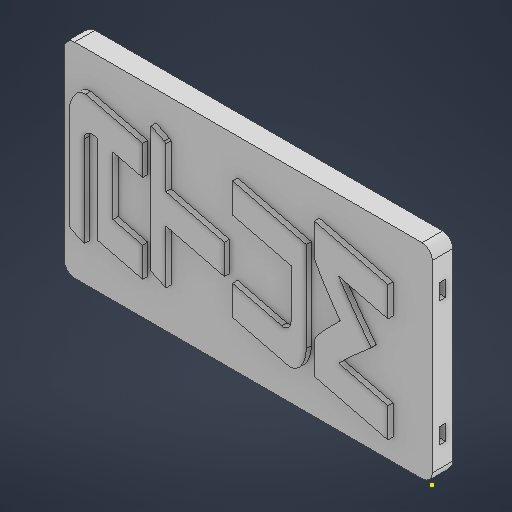
# Autodesk Inventor part: custom  plate vertical
Saved by Autodesk Inventor 2025.1 (Build 291241000, 241)
## iProperties
Created: 2024-12-05
Part Number: custom  plate vertical
Material: Generic
Document SubType Name: Modeling
Designer: Hunter Mathis
Density: 1 g/cm^3
Appearance: Default
Author: Hunter Mathis
Autodesk Inventor part; units mm, degrees
ref_plane "YZ Plane" through (0, 0, 0) normal (1, 0, 0) x (0, 1, 0)
ref_plane "XZ Plane" through (0, 0, 0) normal (0, 1, 0) x (-1, 0, 0)
sketch "Sketch1" plane through (0, 0, 0) normal (0, 0, 1) x (1, 0, 0)
  line L0 (0, 0) -> (-114.3, 0)
  line L1 (-114.3, 0) -> (-114.3, 63.5)
  line L2 (-114.3, 63.5) -> (0, 63.5)
  line L3 (0, 63.5) -> (0, 0)
  dimension "d7" = 114.3
  dimension "d8" = 63.5
  constraints: 8 end point, 2 parallel, 1 horizontal, 1 perpendicular
  measures "d7" distance of L1.end L2.end
  measures "d8" distance of L0.end L1.end
extrude "Extrusion1" add sketch "Sketch1" along normal blind 6.35
sketch "Sketch2" plane through (0, 0, 6.35) normal (0, 0, 1) x (1, 0, 0)
  line L0 (0, 0) -> (0, 63.5) projected
  line L1 (-114.3, 63.5) -> (-114.3, 0) projected
  line L2 (-114.3, 0) -> (0, 0) projected
  line L3 (0, 63.5) -> (-114.3, 63.5) projected
sketch "Sketch3" plane through (0, 0, 6.35) normal (0, 0, 1) x (1, 0, 0)
  line L0 (-110.6716, 35.2666) -> (-52.0005, 35.2666) construction
  line L1 (-52.0005, 35.2666) -> (-52.0005, 28.3217) construction
  line L2 (-52.0005, 28.3217) -> (-110.6716, 28.3217) construction
  line L3 (-110.6716, 28.3217) -> (-110.6716, 35.2666) construction
  line L4 (-114.3, 63.5) -> (-114.3, 0) projected
  point P0 (0, 0)
  constraints: 2 other
extrude "Extrusion2" [suppressed]
fillet "Fillet2" radius 3.175 4 edges at (-114.3, 63.5, 3.175) (-114.3, 0, 3.175) (0, 0, 3.175) (0, 63.5, 3.175)
sketch "Sketch4" plane through (0, 0, 6.35) normal (0, 0, 1) x (1, 0, 0)
  point P0 (0, 0)
sketch "Sketch5" plane through (0, 0, 6.35) normal (0, 0, 1) x (1, 0, 0)
  point P0 (0, 0)
sketch "Sketch6" plane through (0, 0, 6.35) normal (0, 0, 1) x (1, 0, 0)
  point P0 (0, 0)
ref_plane "Work Plane1" through (-57.15, 3.175, 0) normal (1, 0, 0) x (0, 0, -1)
sketch "Sketch7" plane through (-111.125, 63.5, 0) normal (0, 1, 0) x (1, 0, 0)
  line L0 (107.95, -6.35) -> (0, -6.35) projected
  line L1 (107.95, 0) -> (0, 0) projected
  line L2 (0, -6.35) -> (0, -3.175)
  line L3 (0, -6.35) -> (0, 0) projected
  line L4 (0, 0) -> (0, -6.35) projected
  line L5 (0, -6.35) -> (0, -3.5306)
  line L6 (0, -3.5306) -> (6.985, -3.5306)
  line L7 (6.985, -3.5306) -> (11.8618, -3.5306)
  line L8 (11.8618, -3.5306) -> (11.8618, -1.651)
  line L9 (11.8618, -1.651) -> (6.985, -1.651)
  line L10 (6.985, -1.651) -> (6.985, -3.5306)
  point P0 (111.125, 0)
  dimension "d24" = 4.8768
  dimension "d25" = 1.8796
  dimension "d26" = 2.8194
  dimension "d27" = 6.985
  constraints: 14 end point, 2 horizontal, 2 parallel, 1 midpoint, 1 perpendicular, 1 point on line
  measures "d24" distance of L6.end L7.end
  measures "d25" distance of L7.end L8.end
  measures "d26" distance between parallel lines of L6 L0
  measures "d27" distance of L5.end L6.end
extrude "Extrusion3" [suppressed]
sketch "Sketch8" plane through (-111.125, 0, 0) normal (0, -1, 0) x (1, 0, 0)
  line L0 (0, 0) -> (0, 6.35) projected
  line L1 (6.985, 3.5306) -> (6.985, 1.651) projected
  line L2 (11.8618, 1.651) -> (11.8618, 3.5306) projected
  line L3 (6.985, 1.651) -> (11.8618, 1.651)
  line L4 (11.8618, 1.651) -> (11.8618, 3.5306)
  line L5 (11.8618, 3.5306) -> (6.985, 3.5306)
  line L6 (6.985, 3.5306) -> (6.985, 1.651)
  line L7 (0, 0) -> (107.95, 0) projected
  point P0 (111.125, 0)
  constraints: 8 end point, 2 parallel, 1 horizontal, 1 perpendicular
extrude "Extrusion4" [suppressed]
mirror "Mirror1" [suppressed]
mirror "Mirror2" [suppressed]
sketch "Sketch9" plane through (0, 0, 6.35) normal (0, 0, 1) x (1, 0, 0)
  point P0 (0, 0)
sketch "Sketch10" plane through (0, 0, 6.35) normal (0, 0, 1) x (1, 0, 0)
  line L0 (-111.2518, 27.0157) -> (-111.2518, 30.2464) construction
  line L1 (-111.2518, 30.2464) -> (-93.1484, 30.2464) construction
  line L2 (-93.1484, 30.2464) -> (-93.1484, 27.0157) construction
  line L3 (-93.1484, 27.0157) -> (-111.2518, 27.0157) construction
  line L4 (-114.3, 60.325) -> (-114.3, 3.175) projected
  line L5 (-114.3, 60.325) -> (-114.3, 3.175)
  line L6 (-114.3, 3.175) -> (-114.3, 31.75)
  line L7 (0, 3.175) -> (0, 60.325) projected
  line L8 (-88.3918, 11.8288) -> (-102.3042, 15.3115)
  line L9 (-102.3042, 15.3115) -> (-102.3042, 42.6731)
  line L10 (-102.3042, 42.6731) -> (-103.638, 42.988)
  spline S0 degree 2 poles (-103.638, 42.988) (-104.2308, 43.1362) (-105.2867, 42.8213) (-106.0833, 42.1173) (-106.5464, 41.0799) (-106.5464, 40.5242) knots 0 0 0 1 2 3 4 4 4
  line L11 (-106.5464, 40.5242) -> (-106.5464, 12.3845)
  spline S1 degree 2 poles (-106.5464, 12.3845) (-107.4912, 12.8106) (-109.7327, 13.8295) (-110.6775, 14.3297) knots 0 0 0 1 2 2 2
  line L12 (-110.6775, 14.3297) -> (-111.2518, 14.7743)
  line L13 (-111.2518, 14.7743) -> (-111.2518, 45.3222)
  spline S2 degree 2 poles (-111.2518, 45.3222) (-111.2518, 46.5078) (-110.6034, 49.1569) (-109.2881, 51.3984) (-107.38, 52.8434) (-106.0648, 52.8063) knots 0 0 0 1 2 3 4 4 4
  line L14 (-106.0648, 52.8063) -> (-88.3918, 48.3974)
  line L15 (-88.3918, 48.3974) -> (-88.3918, 39.1904)
  line L16 (-88.3918, 39.1904) -> (-97.5988, 41.469)
  line L17 (-97.5988, 41.469) -> (-97.5988, 23.3143)
  line L18 (-97.5988, 23.3143) -> (-88.3918, 21.0358)
  line L19 (-88.3918, 21.0358) -> (-88.3918, 11.8288)
  spline S3 degree 2 poles (-81.1464, 13.144) (-82.0912, 13.5701) (-84.3327, 14.589) (-85.2775, 15.0892) knots 0 0 0 1 2 2 2
  line L20 (-85.2775, 15.0892) -> (-85.8518, 15.5338)
  line L21 (-85.8518, 15.5338) -> (-85.8518, 54.3439)
  spline S4 degree 2 poles (-85.8518, 54.3439) (-84.907, 53.9734) (-82.6655, 52.9175) (-81.7207, 52.3803) knots 0 0 0 1 2 2 2
  line L22 (-81.7207, 52.3803) -> (-81.1464, 51.9357)
  line L23 (-81.1464, 51.9357) -> (-81.1464, 39.0051)
  line L24 (-81.1464, 39.0051) -> (-62.9918, 34.485)
  line L25 (-62.9918, 34.485) -> (-62.9918, 25.278)
  line L26 (-62.9918, 25.278) -> (-81.1464, 29.7981)
  line L27 (-81.1464, 29.7981) -> (-81.1464, 13.144)
  spline S5 degree 2 poles (-42.7788, 11.1619) (-41.4635, 11.1248) (-39.5555, 12.5512) (-38.2402, 14.7928) (-37.5918, 17.4419) (-37.5918, 18.6275) knots 0 0 0 1 2 3 4 4 4
  line L28 (-37.5918, 18.6275) -> (-37.5918, 46.6004)
  line L29 (-37.5918, 46.6004) -> (-60.4518, 52.2876)
  line L30 (-60.4518, 52.2876) -> (-60.4518, 43.0806)
  line L31 (-60.4518, 43.0806) -> (-42.2972, 38.5605)
  line L32 (-42.2972, 38.5605) -> (-42.2972, 23.407)
  spline S6 degree 2 poles (-42.2972, 23.407) (-42.2972, 22.8697) (-42.7603, 21.8509) (-43.5569, 21.1284) (-44.6128, 20.8134) (-45.1871, 20.9431) knots 0 0 0 1 2 3 4 4 4
  line L33 (-45.1871, 20.9431) -> (-60.4518, 24.7593)
  line L34 (-60.4518, 24.7593) -> (-60.4518, 15.5523)
  line L35 (-60.4518, 15.5523) -> (-42.7788, 11.1619)
  line L36 (-35.0518, 12.403) -> (-12.1918, 6.7158)
  line L37 (-12.1918, 6.7158) -> (-12.1918, 15.9228)
  line L38 (-12.1918, 15.9228) -> (-27.475, 19.7205)
  spline S7 degree 2 poles (-27.475, 19.7205) (-26.5302, 20.7393) (-24.1775, 22.9809) (-21.5655, 25.3336) (-18.8238, 27.6863) (-17.4715, 28.8534) knots 0 0 0 1 2 3 4 4 4
  line L39 (-17.4715, 28.8534) -> (-17.4715, 28.9645)
  spline S8 degree 2 poles (-17.4715, 28.9645) (-18.8238, 30.78) (-21.6026, 34.5406) (-24.2146, 38.1715) (-26.5302, 41.5986) (-27.475, 43.0992) knots 0 0 0 1 2 3 4 4 4
  line L40 (-27.475, 43.0992) -> (-12.1918, 39.283)
  line L41 (-12.1918, 39.283) -> (-12.1918, 48.49)
  line L42 (-12.1918, 48.49) -> (-35.0518, 54.1772)
  line L43 (-35.0518, 54.1772) -> (-35.0518, 44.2107)
  spline S9 degree 2 poles (-35.0518, 44.2107) (-34.5146, 43.0621) (-33.014, 40.376) (-31.2171, 37.5046) (-29.2164, 34.5406) (-28.1975, 33.0215) knots 0 0 0 1 2 3 4 4 4
  line L44 (-28.1975, 33.0215) -> (-27.0489, 31.2801)
  spline S10 degree 2 poles (-27.0489, 31.2801) (-29.9759, 28.4087) (-33.9959, 24.2221) (-35.0518, 22.3696) knots 0 0 0 1 2 2 2
  line L45 (-35.0518, 22.3696) -> (-35.0518, 12.403)
  point P0 (0, 0)
  constraints: 4 end point, 1 collinear, 1 midpoint, 2 other
sketch "Sketch11" plane through (0, 3.175, 0) normal (1, 0, 0) x (0, 0, -1)
  line L0 (0, 0) -> (-6.35, 0) projected
  line L1 (-3.175, 0) -> (-3.175, 8.89)
  line L2 (-4.1148, 6.4516) -> (-2.2352, 6.4516)
  line L3 (-2.2352, 6.4516) -> (-2.2352, 11.3284)
  line L4 (-2.2352, 11.3284) -> (-4.1148, 11.3284)
  line L5 (-4.1148, 11.3284) -> (-4.1148, 6.4516)
  line L6 (-4.1148, 6.4516) -> (-2.2352, 11.3284) construction
  line L7 (-2.2352, 6.4516) -> (-4.1148, 11.3284) construction
  line L8 (0, 60.325) -> (-6.35, 60.325) projected
  line L9 (-3.175, 60.325) -> (-3.175, 47.625)
  line L10 (-4.1148, 45.1866) -> (-2.2352, 45.1866)
  line L11 (-2.2352, 45.1866) -> (-2.2352, 50.0634)
  line L12 (-2.2352, 50.0634) -> (-4.1148, 50.0634)
  line L13 (-4.1148, 50.0634) -> (-4.1148, 45.1866)
  line L14 (-4.1148, 45.1866) -> (-2.2352, 50.0634) construction
  line L15 (-2.2352, 45.1866) -> (-4.1148, 50.0634) construction
  point P0 (0, -3.175)
  point P1 (-2.2352, 47.625)
  dimension "d29" = 8.89
  dimension "d30" = 12.7
  dimension "d31" = 4.8768
  dimension "d32" = 1.8796
  dimension "d33" = 4.8768
  dimension "d34" = 1.8796
  constraints: 28 end point, 7 midpoint, 4 parallel, 2 horizontal, 2 perpendicular, 2 vertical
  measures "d29" distance of L1.start L1.end
  measures "d30" distance of L9.start L9.end
  measures "d31" distance between parallel lines of L12 L10
  measures "d32" distance from line of point (-2.235, 47.625) L13
  measures "d33" distance between parallel lines of L4 L2
  measures "d34" distance between parallel lines of L3 L5
extrude "Extrusion5" cut sketch "Sketch11" against normal blind 9.652
extrude "Extrusion6" add sketch "Sketch10" along normal blind 1.5875
body "Solid1"
